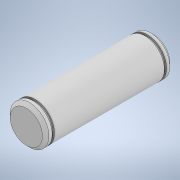
# Autodesk Inventor part: Pin til stang
Saved by Autodesk Inventor 2022 (Build 260153000, 153)
## iProperties
Created: 2022-04-12
Part Number: Pin til stang
Material: Generic
Document SubType Name: Modeling
Designer: Patrick
Density: 1 g/cm^3
Appearance: Default
Author: Patrick
Autodesk Inventor part; units mm, degrees
ref_plane "YZ Plane" through (0, 0, 0) normal (1, 0, 0) x (0, 1, 0)
ref_plane "XZ Plane" through (0, 0, 0) normal (0, 1, 0) x (-1, 0, 0)
ref_plane "XY Plane" through (0, 0, 0) normal (0, 0, 1) x (1, 0, 0)
sketch "Sketch1" plane through (0, 0, 0) normal (0, 1, 0) x (-1, 0, 0)
  line L0 (0, 0) -> (6, 0)
  line L1 (6, 0) -> (6, -17)
  line L2 (6, -17) -> (5.5, -17)
  line L3 (5.5, -17) -> (5.5, -17.7)
  line L4 (0, -19.7) -> (0, 0)
  line L5 (5.5, -17.7) -> (6, -17.7)
  line L6 (6, -17.7) -> (6, -18.7)
  line L7 (0, -19.7) -> (5, -19.7)
  line L8 (6, -18.7) -> (5, -19.7)
  line L9 (6, 0) -> (6, 17)
  line L10 (6, 17) -> (5.5, 17)
  line L11 (5.5, 17) -> (5.5, 17.7)
  line L12 (0, 19.7) -> (0, 0)
  line L13 (5.5, 17.7) -> (6, 17.7)
  line L14 (6, 17.7) -> (6, 18.7)
  line L15 (0, 19.7) -> (5, 19.7)
  line L16 (6, 18.7) -> (5, 19.7)
  point P0 (6, -19.7)
  dimension "d0" = 6
  dimension "d1" = 17
  dimension "d2" = 0.7
  dimension "d3" = 0.5
  dimension "d7" = 2
  dimension "d8" = 1
  dimension "d9" = 1
  constraints: 34 end point, 7 symmetric about line, 5 perpendicular, 2 horizontal, 2 point on line, 1 collinear
  measures "d0" distance between parallel lines of L4 L1
  measures "d1" distance between parallel lines of L0 L2
  measures "d2" distance of L2.end L3.end
  measures "d3" distance of L1.end L2.end
  measures "d7" distance between parallel lines of L5 L7
  measures "d8" distance of L6.end point (6, -19.7)
  measures "d9" distance of L7.end point (6, -19.7)
revolve "Revolution1" add sketch "Sketch1" angle 360 about axis through (0, 0, 19.7) along (0, 0, -1)
equation "\"d9\" = d8"
body "Solid1"
